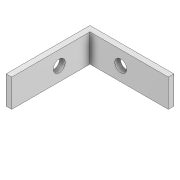
# Autodesk Inventor part: esquina de bandeja
Saved by Autodesk Inventor 2020.3 (Build 243373000, 373)
## iProperties
Created: 2020-06-07
Part Number: esquina de bandeja
Material: Aluminum 1100-H14
Document SubType Name: Modeling
Designer: Pipi
Density: 2.7 g/cm^3
Appearance: Satin
Author: Pipi
Autodesk Inventor part; units mm, degrees
ref_plane "YZ Plane" through (0, 0, 0) normal (1, 0, 0) x (0, 1, 0)
ref_plane "XZ Plane" through (0, 0, 0) normal (0, 1, 0) x (-1, 0, 0)
ref_plane "XY Plane" through (0, 0, 0) normal (0, 0, 1) x (1, 0, 0)
sketch "Boceto1" plane through (0, 0, 0) normal (0, 1, 0) x (-1, 0, 0)
  line L0 (4.3845, 19.6649) -> (4.3845, -10.3351)
  line L1 (4.3845, -10.3351) -> (-25.6155, -10.3351)
  line L2 (-25.6155, -10.3351) -> (-25.6155, -8.3351)
  line L3 (-25.6155, -8.3351) -> (2.3845, -8.3351)
  line L4 (2.3845, -8.3351) -> (2.3845, 19.6649)
  line L5 (2.3845, 19.6649) -> (4.3845, 19.6649)
  point P0 (0, 0)
  dimension "d0" = 30
  dimension "d1" = 30
  dimension "d2" = 2
  dimension "d3" = 28
  constraints: 12 end point, 5 perpendicular, 1 vertical
  measures "d0" distance of L0.start L0.end
  measures "d1" distance of L0.end L1.end
  measures "d2" distance of L1.end L2.end
  measures "d3" distance of L2.end L3.end
extrude "Extrusión1" add sketch "Boceto1" along normal blind 10
sketch "Boceto2" plane through (-2.3845, 0, 19.6649) normal (1, 0, 0) x (0, 0, -1)
  line L0 (0, 0) -> (0, 10) projected
  circle A0 centre (17, 5) radius 2.125
  line L1 (28, 0) -> (28, 10) projected
  line L2 (28, 10) -> (28, 2.875)
  point P0 (19.6649, 0)
  dimension "d6" = 4.25
  dimension "d7" = 17
  constraints: 2 end point, 1 centre point, 1 point on line
  measures "d6" diameter of A0
  measures "d7" distance from line of A0.centre L0
extrude "Extrusión2" cut sketch "Boceto2" against normal blind 10
sketch "Boceto3" plane through (-2.3845, 0, -8.3351) normal (0, 0, 1) x (1, 0, 0)
  line L0 (28, 0) -> (28, 10) projected
  circle A0 centre (11, 5) radius 2.125
  point P0 (2.3845, 0)
  dimension "d10" = 4.25
  dimension "d11" = 17
  constraints: 1 centre point
  measures "d10" diameter of A0
  measures "d11" distance from line of L0 A0.centre
extrude "Extrusión3" cut sketch "Boceto3" against normal blind 10
